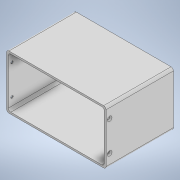
# Autodesk Inventor part: battery case
Saved by Autodesk Inventor 2021 (Build 250183000, 183)
## iProperties
Created: 2022-01-29
Part Number: battery case
Material: Generic
Document SubType Name: Modeling
Designer: Toby
Density: 1 g/cm^3
Appearance: Default
Author: Toby
Autodesk Inventor part; units mm, degrees
ref_plane "YZ Plane" through (0, 0, 0) normal (1, 0, 0) x (0, 1, 0)
ref_plane "XZ Plane" through (0, 0, 0) normal (0, 1, 0) x (-1, 0, 0)
ref_plane "XY Plane" through (0, 0, 0) normal (0, 0, 1) x (1, 0, 0)
sketch "Sketch1" plane through (0, 0, 0) normal (0, 0, 1) x (1, 0, 0)
  line L0 (-60.7718, 21.5285) -> (19.2282, 21.5285)
  line L1 (19.2282, 21.5285) -> (19.2282, -20.4715)
  line L2 (19.2282, -20.4715) -> (-60.7718, -20.4715)
  line L3 (-60.7718, -20.4715) -> (-60.7718, 21.5285)
  line L4 (-62.2718, 23.0285) -> (20.7282, 23.0285)
  line L5 (20.7282, 23.0285) -> (20.7282, -21.9715)
  line L6 (20.7282, -21.9715) -> (-62.2718, -21.9715)
  line L7 (-62.2718, -21.9715) -> (-62.2718, 23.0285)
  point P0 (0, 0)
  dimension "d0" = 80
  dimension "d1" = 42
  dimension "d2" = 1.5
  dimension "d3" = 1.5
  dimension "d4" = 1.5
  dimension "d5" = 1.5
  constraints: 16 end point, 4 parallel, 2 horizontal, 2 perpendicular
  measures "d0" distance of L0.start L0.end
  measures "d1" distance of L2.end L0.start
  measures "d2" distance between parallel lines of L0 L4
  measures "d3" distance between parallel lines of L6 L2
  measures "d4" distance between parallel lines of L7 L3
  measures "d5" distance between parallel lines of L5 L1
extrude "Extrusion1" add sketch "Sketch1" along normal blind 55
sketch "Sketch2" plane through (0, 0, 0) normal (0, 0, -1) x (-1, 0, 0)
  line L0 (-20.7282, 23.0285) -> (62.2718, 23.0285) projected
  line L1 (62.2718, -21.9715) -> (-20.7282, -21.9715) projected
  line L2 (-20.7282, 23.0285) -> (62.2718, 23.0285)
  line L3 (62.2718, 23.0285) -> (62.2718, -21.9715)
  line L4 (62.2718, -21.9715) -> (-20.7282, -21.9715)
  line L5 (-20.7282, -21.9715) -> (-20.7282, 23.0285)
  point P0 (0, 0)
  point P1 (62.2718, 23.0285)
  constraints: 8 end point, 2 parallel, 1 horizontal, 1 perpendicular
extrude "Extrusion2" add sketch "Sketch2" along normal blind 1.2
sketch "Sketch3" plane through (-62.2718, -21.9715, 55) normal (-1, 0, 0) x (0, 0, 1)
  line L0 (-40, 27) -> (-44, 27)
  line L1 (-44, 27) -> (-44, 18)
  line L2 (-44, 18) -> (-40, 18)
  line L3 (-40, 18) -> (-40, 27)
  line L4 (-55, 1.5) -> (-55, 43.5) projected
  line L5 (-55, 1.5) -> (0, 1.5) projected
  line L6 (-55, 43.5) -> (0, 43.5) projected
  point P0 (-55, 21.9715)
  dimension "d10" = 11
  dimension "d11" = 15
  dimension "d12" = 9
  dimension "d13" = 16.5
  dimension "d14" = 16.5
  constraints: 8 end point, 2 parallel, 1 horizontal, 1 perpendicular
  measures "d10" distance between parallel lines of L4 L1
  measures "d11" distance between parallel lines of L4 L3
  measures "d12" distance between parallel lines of L2 L0
  measures "d13" distance between parallel lines of L5 L2
  measures "d14" distance between parallel lines of L6 L0
extrude "Extrusion3" cut sketch "Sketch3" against normal blind 2
chamfer "Chamfer1" distance 1.5 angle 45 4 edges at (-62.2718, 0.5285, 15) (-62.2718, 0.5285, 11) (-62.2718, 5.0285, 13) (-62.2718, -3.9715, 13)
sketch "Sketch4" plane through (-62.2718, -21.9715, 55) normal (0, -1, 0) x (1, 0, 0)
  line L0 (58.5, -52) -> (78.5, -52)
  line L1 (78.5, -52) -> (78.5, -37)
  line L2 (78.5, -37) -> (58.5, -37)
  line L3 (58.5, -37) -> (58.5, -52)
  line L4 (81.5, -55) -> (1.5, -55) projected
  line L5 (81.5, -55) -> (81.5, 0) projected
  point P0 (62.2718, -55)
  dimension "d20" = 3
  dimension "d21" = 3
  dimension "d22" = 20
  dimension "d23" = 15
  constraints: 8 end point, 2 parallel, 1 horizontal, 1 perpendicular
  measures "d20" distance between parallel lines of L4 L0
  measures "d21" distance between parallel lines of L5 L1
  measures "d22" distance of L1.end L2.end
  measures "d23" distance of L2.end L0.start
extrude "Extrusion4" cut sketch "Sketch4" against normal blind 2
fillet "Fillet1" radius 2 8 edges at (19.2282, 21.5285, 27.5) (20.7282, 23.0285, 26.9) (19.2282, -20.4715, 27.5) (20.7282, -21.9715, 26.9) (-60.7718, -20.4715, 27.5) (-62.2718, -21.9715, 26.9) (-60.7718, 21.5285, 27.5) (-62.2718, 23.0285, 26.9)
sketch "Sketch5" plane through (-62.2718, -19.9715, -1.2) normal (-1, 0, 0) x (0, 0, 1)
  line L0 (56.2, 41) -> (56.2, 0) projected
  line L1 (0, -2) -> (56.2, -2) projected
  line L2 (56.2, 43) -> (0, 43) projected
  point P0 (1.2, 19.9715)
  point P1 (53.2, 8)
  point P2 (53.2, 33)
  dimension "d27" = 3
  dimension "d28" = 3
  dimension "d29" = 10
  dimension "d30" = 10
  measures "d27" distance from line of L0 point (53.2, 8)
  measures "d28" distance from line of L0 point (53.2, 33)
  measures "d29" distance from line of L1 point (53.2, 8)
  measures "d30" distance from line of L2 point (53.2, 33)
hole "Hole1" at (-62.2718, -11.9715, 52) at (-62.2718, 13.0285, 52) direction (1, 0, 0) diameter 2 depth 10 tip angle 179 countersink diameter 4 countersink angle 90
sketch "Sketch6" plane through (20.7282, -19.9715, -1.2) normal (1, 0, 0) x (0, 0, -1)
  circle A0 centre (-53.2, 33) radius 1 projected
  circle A1 centre (-53.2, 8) radius 1 projected
  point P0 (-1.2, 19.9715)
  constraints: 2 coincident
hole "Hole2" at (20.7282, 13.0285, 52) at (20.7282, -11.9715, 52) direction (-1, 0, 0) diameter 2 depth 10 tip angle 179 countersink diameter 4 countersink angle 90
body "Solid1"
